Autodesk Fusion 360 part; units mm, degrees
(part 2 of 4)
  line L565 (-143.125, 35.2707) -> (-143.125, 31.2293)
  line L566 (-143.125, 31.2293) -> (-139.625, 29.2085)
  line L567 (-136.125, 31.2293) -> (-136.125, 35.2707)
  line L568 (-152.125, 31.2293) -> (-148.625, 29.2085)
  line L569 (-122.625, 43.065) -> (-126.125, 45.0857)
  line L570 (-126.125, 45.0857) -> (-129.625, 43.065)
  line L571 (-122.625, 39.0235) -> (-122.625, 43.065)
  line L572 (-134.125, 35.2707) -> (-134.125, 31.2293)
  line L573 (-127.125, 31.2293) -> (-127.125, 35.2707)
  line L574 (-129.625, 39.0235) -> (-126.125, 37.0028)
  line L575 (-135.125, 45.0857) -> (-138.625, 43.065)
  line L576 (-131.625, 39.0235) -> (-131.625, 43.065)
  line L577 (-130.625, 37.2915) -> (-134.125, 35.2707)
  line L578 (-130.625, 29.2085) -> (-127.125, 31.2293)
  line L579 (-131.625, 43.065) -> (-135.125, 45.0857)
  line L580 (-138.625, 39.0235) -> (-135.125, 37.0028)
  line L581 (-135.125, 37.0028) -> (-131.625, 39.0235)
  line L582 (-127.125, 35.2707) -> (-130.625, 37.2915)
  line L583 (-129.625, 43.065) -> (-129.625, 39.0235)
  line L584 (-138.625, 43.065) -> (-138.625, 39.0235)
  line L585 (-126.125, 37.0028) -> (-122.625, 39.0235)
  line L586 (-121.625, 37.2915) -> (-125.125, 35.2707)
  line L587 (-118.125, 35.2707) -> (-121.625, 37.2915)
  line L588 (-121.625, 29.2085) -> (-118.125, 31.2293)
  line L589 (-125.125, 35.2707) -> (-125.125, 31.2293)
  line L590 (-125.125, 31.2293) -> (-121.625, 29.2085)
  line L591 (-118.125, 31.2293) -> (-118.125, 35.2707)
  line L592 (-134.125, 31.2293) -> (-130.625, 29.2085)
  line L593 (-104.625, 43.065) -> (-108.125, 45.0857)
  line L594 (-108.125, 45.0857) -> (-111.625, 43.065)
  line L595 (-104.625, 39.0235) -> (-104.625, 43.065)
  line L596 (-116.125, 35.2707) -> (-116.125, 31.2293)
  line L597 (-109.125, 31.2293) -> (-109.125, 35.2707)
  line L598 (-111.625, 39.0235) -> (-108.125, 37.0028)
  line L599 (-117.125, 45.0857) -> (-120.625, 43.065)
  line L600 (-113.625, 39.0235) -> (-113.625, 43.065)
  line L601 (-112.625, 37.2915) -> (-116.125, 35.2707)
  line L602 (-112.625, 29.2085) -> (-109.125, 31.2293)
  line L603 (-113.625, 43.065) -> (-117.125, 45.0857)
  line L604 (-120.625, 39.0235) -> (-117.125, 37.0028)
  line L605 (-117.125, 37.0028) -> (-113.625, 39.0235)
  line L606 (-109.125, 35.2707) -> (-112.625, 37.2915)
  line L607 (-111.625, 43.065) -> (-111.625, 39.0235)
  line L608 (-120.625, 43.065) -> (-120.625, 39.0235)
  line L609 (-108.125, 37.0028) -> (-104.625, 39.0235)
  line L610 (-103.625, 37.2915) -> (-107.125, 35.2707)
  line L611 (-100.125, 35.2707) -> (-103.625, 37.2915)
  line L612 (-103.625, 29.2085) -> (-100.125, 31.2293)
  line L613 (-107.125, 35.2707) -> (-107.125, 31.2293)
  line L614 (-107.125, 31.2293) -> (-103.625, 29.2085)
  line L615 (-100.125, 31.2293) -> (-100.125, 35.2707)
  line L616 (-116.125, 31.2293) -> (-112.625, 29.2085)
  line L617 (-86.625, 43.065) -> (-90.125, 45.0857)
  line L618 (-90.125, 45.0857) -> (-93.625, 43.065)
  line L619 (-86.625, 39.0235) -> (-86.625, 43.065)
  line L620 (-98.125, 35.2707) -> (-98.125, 31.2293)
  line L621 (-91.125, 31.2293) -> (-91.125, 35.2707)
  line L622 (-93.625, 39.0235) -> (-90.125, 37.0028)
  line L623 (-99.125, 45.0857) -> (-102.625, 43.065)
  line L624 (-95.625, 39.0235) -> (-95.625, 43.065)
  line L625 (-94.625, 37.2915) -> (-98.125, 35.2707)
  line L626 (-94.625, 29.2085) -> (-91.125, 31.2293)
  line L627 (-95.625, 43.065) -> (-99.125, 45.0857)
  line L628 (-102.625, 39.0235) -> (-99.125, 37.0028)
  line L629 (-99.125, 37.0028) -> (-95.625, 39.0235)
  line L630 (-91.125, 35.2707) -> (-94.625, 37.2915)
  line L631 (-93.625, 43.065) -> (-93.625, 39.0235)
  line L632 (-102.625, 43.065) -> (-102.625, 39.0235)
  line L633 (-90.125, 37.0028) -> (-86.625, 39.0235)
  line L634 (-85.625, 37.2915) -> (-89.125, 35.2707)
  line L635 (-82.125, 35.2707) -> (-85.625, 37.2915)
  line L636 (-85.625, 29.2085) -> (-82.125, 31.2293)
  line L637 (-89.125, 35.2707) -> (-89.125, 31.2293)
  line L638 (-89.125, 31.2293) -> (-85.625, 29.2085)
  line L639 (-82.125, 31.2293) -> (-82.125, 35.2707)
  line L640 (-98.125, 31.2293) -> (-94.625, 29.2085)
  line L641 (-50.625, 43.065) -> (-54.125, 45.0857)
  line L642 (-54.125, 45.0857) -> (-57.625, 43.065)
  line L643 (-50.625, 39.0235) -> (-50.625, 43.065)
  line L644 (-62.125, 35.2707) -> (-62.125, 31.2293)
  line L645 (-55.125, 31.2293) -> (-55.125, 35.2707)
  line L646 (-57.625, 39.0235) -> (-54.125, 37.0028)
  line L647 (-63.125, 45.0857) -> (-66.625, 43.065)
  line L648 (-59.625, 39.0235) -> (-59.625, 43.065)
  line L649 (-58.625, 37.2915) -> (-62.125, 35.2707)
  line L650 (-58.625, 29.2085) -> (-55.125, 31.2293)
  line L651 (-59.625, 43.065) -> (-63.125, 45.0857)
  line L652 (-66.625, 39.0235) -> (-63.125, 37.0028)
  line L653 (-63.125, 37.0028) -> (-59.625, 39.0235)
  line L654 (-55.125, 35.2707) -> (-58.625, 37.2915)
  line L655 (-57.625, 43.065) -> (-57.625, 39.0235)
  line L656 (-66.625, 43.065) -> (-66.625, 39.0235)
  line L657 (-54.125, 37.0028) -> (-50.625, 39.0235)
  line L658 (-49.625, 37.2915) -> (-53.125, 35.2707)
  line L659 (-46.125, 35.2707) -> (-49.625, 37.2915)
  line L660 (-49.625, 29.2085) -> (-46.125, 31.2293)
  line L661 (-53.125, 35.2707) -> (-53.125, 31.2293)
  line L662 (-53.125, 31.2293) -> (-49.625, 29.2085)
  line L663 (-46.125, 31.2293) -> (-46.125, 35.2707)
  line L664 (-62.125, 31.2293) -> (-58.625, 29.2085)
  line L665 (-32.625, 43.065) -> (-36.125, 45.0857)
  line L666 (-36.125, 45.0857) -> (-39.625, 43.065)
  line L667 (-32.625, 39.0235) -> (-32.625, 43.065)
  line L668 (-44.125, 35.2707) -> (-44.125, 31.2293)
  line L669 (-37.125, 31.2293) -> (-37.125, 35.2707)
  line L670 (-39.625, 39.0235) -> (-36.125, 37.0028)
  line L671 (-45.125, 45.0857) -> (-48.625, 43.065)
  line L672 (-41.625, 39.0235) -> (-41.625, 43.065)
  line L673 (-40.625, 37.2915) -> (-44.125, 35.2707)
  line L674 (-40.625, 29.2085) -> (-37.125, 31.2293)
  line L675 (-41.625, 43.065) -> (-45.125, 45.0857)
  line L676 (-48.625, 39.0235) -> (-45.125, 37.0028)
  line L677 (-45.125, 37.0028) -> (-41.625, 39.0235)
  line L678 (-37.125, 35.2707) -> (-40.625, 37.2915)
  line L679 (-39.625, 43.065) -> (-39.625, 39.0235)
  line L680 (-48.625, 43.065) -> (-48.625, 39.0235)
  line L681 (-36.125, 37.0028) -> (-32.625, 39.0235)
  line L682 (-31.625, 37.2915) -> (-35.125, 35.2707)
  line L683 (-28.125, 35.2707) -> (-31.625, 37.2915)
  line L684 (-31.625, 29.2085) -> (-28.125, 31.2293)
  line L685 (-35.125, 35.2707) -> (-35.125, 31.2293)
  line L686 (-35.125, 31.2293) -> (-31.625, 29.2085)
  line L687 (-28.125, 31.2293) -> (-28.125, 35.2707)
  line L688 (-44.125, 31.2293) -> (-40.625, 29.2085)
  line L689 (-14.625, 43.065) -> (-18.125, 45.0857)
  line L690 (-18.125, 45.0857) -> (-21.625, 43.065)
  line L691 (-14.625, 39.0235) -> (-14.625, 43.065)
  line L692 (-26.125, 35.2707) -> (-26.125, 31.2293)
  line L693 (-19.125, 31.2293) -> (-19.125, 35.2707)
  line L694 (-21.625, 39.0235) -> (-18.125, 37.0028)
  line L695 (-27.125, 45.0857) -> (-30.625, 43.065)
  line L696 (-23.625, 39.0235) -> (-23.625, 43.065)
  line L697 (-22.625, 37.2915) -> (-26.125, 35.2707)
  line L698 (-22.625, 29.2085) -> (-19.125, 31.2293)
  line L699 (-23.625, 43.065) -> (-27.125, 45.0857)
  line L700 (-30.625, 39.0235) -> (-27.125, 37.0028)
  line L701 (-27.125, 37.0028) -> (-23.625, 39.0235)
  line L702 (-19.125, 35.2707) -> (-22.625, 37.2915)
  line L703 (-21.625, 43.065) -> (-21.625, 39.0235)
  line L704 (-30.625, 43.065) -> (-30.625, 39.0235)
  line L705 (-18.125, 37.0028) -> (-14.625, 39.0235)
  line L706 (-13.625, 37.2915) -> (-17.125, 35.2707)
  line L707 (-10.125, 35.2707) -> (-13.625, 37.2915)
  line L708 (-13.625, 29.2085) -> (-10.125, 31.2293)
  line L709 (-17.125, 35.2707) -> (-17.125, 31.2293)
  line L710 (-17.125, 31.2293) -> (-13.625, 29.2085)
  line L711 (-10.125, 31.2293) -> (-10.125, 35.2707)
  line L712 (-26.125, 31.2293) -> (-22.625, 29.2085)
  line L713 (3.375, 43.065) -> (-0.125, 45.0857)
  line L714 (-0.125, 45.0857) -> (-3.625, 43.065)
  line L715 (3.375, 39.0235) -> (3.375, 43.065)
  line L716 (-8.125, 35.2707) -> (-8.125, 31.2293)
  line L717 (-1.125, 31.2293) -> (-1.125, 35.2707)
  line L718 (-3.625, 39.0235) -> (-0.125, 37.0028)
  line L719 (-9.125, 45.0857) -> (-12.625, 43.065)
  line L720 (-5.625, 39.0235) -> (-5.625, 43.065)
  line L721 (-4.625, 37.2915) -> (-8.125, 35.2707)
  line L722 (-4.625, 29.2085) -> (-1.125, 31.2293)
  line L723 (-5.625, 43.065) -> (-9.125, 45.0857)
  line L724 (-12.625, 39.0235) -> (-9.125, 37.0028)
  line L725 (-9.125, 37.0028) -> (-5.625, 39.0235)
  line L726 (-1.125, 35.2707) -> (-4.625, 37.2915)
  line L727 (-3.625, 43.065) -> (-3.625, 39.0235)
  line L728 (-12.625, 43.065) -> (-12.625, 39.0235)
  line L729 (-0.125, 37.0028) -> (3.375, 39.0235)
  line L730 (4.375, 37.2915) -> (0.875, 35.2707)
  line L731 (7.875, 35.2707) -> (4.375, 37.2915)
  line L732 (4.375, 29.2085) -> (7.875, 31.2293)
  line L733 (0.875, 35.2707) -> (0.875, 31.2293)
  line L734 (0.875, 31.2293) -> (4.375, 29.2085)
  line L735 (7.875, 31.2293) -> (7.875, 35.2707)
  line L736 (-8.125, 31.2293) -> (-4.625, 29.2085)
  line L737 (21.375, 43.065) -> (17.875, 45.0857)
  line L738 (17.875, 45.0857) -> (14.375, 43.065)
  line L739 (21.375, 39.0235) -> (21.375, 43.065)
  line L740 (9.875, 35.2707) -> (9.875, 31.2293)
  line L741 (16.875, 31.2293) -> (16.875, 35.2707)
  line L742 (14.375, 39.0235) -> (17.875, 37.0028)
  line L743 (8.875, 45.0857) -> (5.375, 43.065)
  line L744 (12.375, 39.0235) -> (12.375, 43.065)
  line L745 (13.375, 37.2915) -> (9.875, 35.2707)
  line L746 (13.375, 29.2085) -> (16.875, 31.2293)
  line L747 (12.375, 43.065) -> (8.875, 45.0857)
  line L748 (5.375, 39.0235) -> (8.875, 37.0028)
  line L749 (8.875, 37.0028) -> (12.375, 39.0235)
  line L750 (16.875, 35.2707) -> (13.375, 37.2915)
  line L751 (14.375, 43.065) -> (14.375, 39.0235)
  line L752 (5.375, 43.065) -> (5.375, 39.0235)
  line L753 (17.875, 37.0028) -> (21.375, 39.0235)
  line L754 (22.375, 37.2915) -> (18.875, 35.2707)
  line L755 (25.875, 35.2707) -> (22.375, 37.2915)
  line L756 (22.375, 29.2085) -> (25.875, 31.2293)
  line L757 (18.875, 35.2707) -> (18.875, 31.2293)
  line L758 (18.875, 31.2293) -> (22.375, 29.2085)
  line L759 (25.875, 31.2293) -> (25.875, 35.2707)
  line L760 (9.875, 31.2293) -> (13.375, 29.2085)
  line L761 (-140.625, 58.942) -> (-144.125, 60.9627)
  line L762 (-144.125, 60.9627) -> (-147.625, 58.942)
  line L763 (-140.625, 54.9005) -> (-140.625, 58.942)
  line L764 (-152.125, 51.1477) -> (-152.125, 47.1063)
  line L765 (-145.125, 47.1063) -> (-145.125, 51.1477)
  line L766 (-147.625, 54.9005) -> (-144.125, 52.8798)
  line L767 (-153.125, 60.9627) -> (-156.625, 58.942)
  line L768 (-149.625, 54.9005) -> (-149.625, 58.942)
  line L769 (-148.625, 53.1685) -> (-152.125, 51.1477)
  line L770 (-148.625, 45.0855) -> (-145.125, 47.1063)
  line L771 (-149.625, 58.942) -> (-153.125, 60.9627)
  line L772 (-156.625, 54.9005) -> (-153.125, 52.8798)
  line L773 (-153.125, 52.8798) -> (-149.625, 54.9005)
  line L774 (-145.125, 51.1477) -> (-148.625, 53.1685)
  line L775 (-147.625, 58.942) -> (-147.625, 54.9005)
  line L776 (-156.625, 58.942) -> (-156.625, 54.9005)
  line L777 (-144.125, 52.8798) -> (-140.625, 54.9005)
  line L778 (-139.625, 53.1685) -> (-143.125, 51.1477)
  line L779 (-136.125, 51.1477) -> (-139.625, 53.1685)
  line L780 (-139.625, 45.0855) -> (-136.125, 47.1063)
  line L781 (-143.125, 51.1477) -> (-143.125, 47.1063)
  line L782 (-143.125, 47.1063) -> (-139.625, 45.0855)
  line L783 (-136.125, 47.1063) -> (-136.125, 51.1477)
  line L784 (-152.125, 47.1063) -> (-148.625, 45.0855)
  line L785 (-122.625, 58.942) -> (-126.125, 60.9627)
  line L786 (-126.125, 60.9627) -> (-129.625, 58.942)
  line L787 (-122.625, 54.9005) -> (-122.625, 58.942)
  line L788 (-134.125, 51.1477) -> (-134.125, 47.1063)
  line L789 (-127.125, 47.1063) -> (-127.125, 51.1477)
  line L790 (-129.625, 54.9005) -> (-126.125, 52.8798)
  line L791 (-135.125, 60.9627) -> (-138.625, 58.942)
  line L792 (-131.625, 54.9005) -> (-131.625, 58.942)
  line L793 (-130.625, 53.1685) -> (-134.125, 51.1477)
  line L794 (-130.625, 45.0855) -> (-127.125, 47.1063)
  line L795 (-131.625, 58.942) -> (-135.125, 60.9627)
  line L796 (-138.625, 54.9005) -> (-135.125, 52.8798)
  line L797 (-135.125, 52.8798) -> (-131.625, 54.9005)
  line L798 (-127.125, 51.1477) -> (-130.625, 53.1685)
  line L799 (-129.625, 58.942) -> (-129.625, 54.9005)
  line L800 (-138.625, 58.942) -> (-138.625, 54.9005)
  line L801 (-126.125, 52.8798) -> (-122.625, 54.9005)
  line L802 (-121.625, 53.1685) -> (-125.125, 51.1477)
  line L803 (-118.125, 51.1477) -> (-121.625, 53.1685)
  line L804 (-121.625, 45.0855) -> (-118.125, 47.1063)
  line L805 (-125.125, 51.1477) -> (-125.125, 47.1063)
  line L806 (-125.125, 47.1063) -> (-121.625, 45.0855)
  line L807 (-118.125, 47.1063) -> (-118.125, 51.1477)
  line L808 (-134.125, 47.1063) -> (-130.625, 45.0855)
  line L809 (-104.625, 58.942) -> (-108.125, 60.9627)
  line L810 (-108.125, 60.9627) -> (-111.625, 58.942)
  line L811 (-104.625, 54.9005) -> (-104.625, 58.942)
  line L812 (-116.125, 51.1477) -> (-116.125, 47.1063)
  line L813 (-109.125, 47.1063) -> (-109.125, 51.1477)
  line L814 (-111.625, 54.9005) -> (-108.125, 52.8798)
  line L815 (-117.125, 60.9627) -> (-120.625, 58.942)
  line L816 (-113.625, 54.9005) -> (-113.625, 58.942)
  line L817 (-112.625, 53.1685) -> (-116.125, 51.1477)
  line L818 (-112.625, 45.0855) -> (-109.125, 47.1063)
  line L819 (-113.625, 58.942) -> (-117.125, 60.9627)
  line L820 (-120.625, 54.9005) -> (-117.125, 52.8798)
  line L821 (-117.125, 52.8798) -> (-113.625, 54.9005)
  line L822 (-109.125, 51.1477) -> (-112.625, 53.1685)
  line L823 (-111.625, 58.942) -> (-111.625, 54.9005)
  line L824 (-120.625, 58.942) -> (-120.625, 54.9005)
  line L825 (-108.125, 52.8798) -> (-104.625, 54.9005)
  line L826 (-103.625, 53.1685) -> (-107.125, 51.1477)
  line L827 (-100.125, 51.1477) -> (-103.625, 53.1685)
  line L828 (-103.625, 45.0855) -> (-100.125, 47.1063)
  line L829 (-107.125, 51.1477) -> (-107.125, 47.1063)
  line L830 (-107.125, 47.1063) -> (-103.625, 45.0855)
  line L831 (-100.125, 47.1063) -> (-100.125, 51.1477)
  line L832 (-116.125, 47.1063) -> (-112.625, 45.0855)
  line L833 (-86.625, 58.942) -> (-90.125, 60.9627)
  line L834 (-90.125, 60.9627) -> (-93.625, 58.942)
  line L835 (-86.625, 54.9005) -> (-86.625, 58.942)
  line L836 (-98.125, 51.1477) -> (-98.125, 47.1063)
  line L837 (-91.125, 47.1063) -> (-91.125, 51.1477)
  line L838 (-93.625, 54.9005) -> (-90.125, 52.8798)
  line L839 (-99.125, 60.9627) -> (-102.625, 58.942)
  line L840 (-95.625, 54.9005) -> (-95.625, 58.942)
  line L841 (-94.625, 53.1685) -> (-98.125, 51.1477)
  line L842 (-94.625, 45.0855) -> (-91.125, 47.1063)
  line L843 (-95.625, 58.942) -> (-99.125, 60.9627)
  line L844 (-102.625, 54.9005) -> (-99.125, 52.8798)
  line L845 (-99.125, 52.8798) -> (-95.625, 54.9005)
  line L846 (-91.125, 51.1477) -> (-94.625, 53.1685)
  line L847 (-93.625, 58.942) -> (-93.625, 54.9005)
  line L848 (-102.625, 58.942) -> (-102.625, 54.9005)
  line L849 (-90.125, 52.8798) -> (-86.625, 54.9005)
  line L850 (-85.625, 53.1685) -> (-89.125, 51.1477)
  line L851 (-82.125, 51.1477) -> (-85.625, 53.1685)
  line L852 (-85.625, 45.0855) -> (-82.125, 47.1063)
  line L853 (-89.125, 51.1477) -> (-89.125, 47.1063)
  line L854 (-89.125, 47.1063) -> (-85.625, 45.0855)
  line L855 (-82.125, 47.1063) -> (-82.125, 51.1477)
  line L856 (-98.125, 47.1063) -> (-94.625, 45.0855)
  line L857 (-68.625, 58.942) -> (-72.125, 60.9627)
  line L858 (-72.125, 60.9627) -> (-75.625, 58.942)
  line L859 (-68.625, 54.9005) -> (-68.625, 58.942)
  line L860 (-80.125, 51.1477) -> (-80.125, 47.1063)
  line L861 (-73.125, 47.1063) -> (-73.125, 51.1477)
  line L862 (-75.625, 54.9005) -> (-72.125, 52.8798)
  line L863 (-81.125, 60.9627) -> (-84.625, 58.942)
  line L864 (-77.625, 54.9005) -> (-77.625, 58.942)
  line L865 (-76.625, 53.1685) -> (-80.125, 51.1477)
  line L866 (-76.625, 45.0855) -> (-73.125, 47.1063)
  line L867 (-77.625, 58.942) -> (-81.125, 60.9627)
  line L868 (-84.625, 54.9005) -> (-81.125, 52.8798)
  line L869 (-81.125, 52.8798) -> (-77.625, 54.9005)
  line L870 (-73.125, 51.1477) -> (-76.625, 53.1685)
  line L871 (-75.625, 58.942) -> (-75.625, 54.9005)
  line L872 (-84.625, 58.942) -> (-84.625, 54.9005)
  line L873 (-72.125, 52.8798) -> (-68.625, 54.9005)
  line L874 (-67.625, 53.1685) -> (-71.125, 51.1477)
  line L875 (-64.125, 51.1477) -> (-67.625, 53.1685)
  line L876 (-67.625, 45.0855) -> (-64.125, 47.1063)
  line L877 (-71.125, 51.1477) -> (-71.125, 47.1063)
  line L878 (-71.125, 47.1063) -> (-67.625, 45.0855)
  line L879 (-64.125, 47.1063) -> (-64.125, 51.1477)
  line L880 (-80.125, 47.1063) -> (-76.625, 45.0855)
  line L881 (-50.625, 58.942) -> (-54.125, 60.9627)
  line L882 (-54.125, 60.9627) -> (-57.625, 58.942)
  line L883 (-50.625, 54.9005) -> (-50.625, 58.942)
  line L884 (-62.125, 51.1477) -> (-62.125, 47.1063)
  line L885 (-55.125, 47.1063) -> (-55.125, 51.1477)
  line L886 (-57.625, 54.9005) -> (-54.125, 52.8798)
  line L887 (-63.125, 60.9627) -> (-66.625, 58.942)
  line L888 (-59.625, 54.9005) -> (-59.625, 58.942)
  line L889 (-58.625, 53.1685) -> (-62.125, 51.1477)
  line L890 (-58.625, 45.0855) -> (-55.125, 47.1063)
  line L891 (-59.625, 58.942) -> (-63.125, 60.9627)
  line L892 (-66.625, 54.9005) -> (-63.125, 52.8798)
  line L893 (-63.125, 52.8798) -> (-59.625, 54.9005)
  line L894 (-55.125, 51.1477) -> (-58.625, 53.1685)
  line L895 (-57.625, 58.942) -> (-57.625, 54.9005)
  line L896 (-66.625, 58.942) -> (-66.625, 54.9005)
  line L897 (-54.125, 52.8798) -> (-50.625, 54.9005)
  line L898 (-49.625, 53.1685) -> (-53.125, 51.1477)
  line L899 (-46.125, 51.1477) -> (-49.625, 53.1685)
  line L900 (-49.625, 45.0855) -> (-46.125, 47.1063)
  line L901 (-53.125, 51.1477) -> (-53.125, 47.1063)
  line L902 (-53.125, 47.1063) -> (-49.625, 45.0855)
  line L903 (-46.125, 47.1063) -> (-46.125, 51.1477)
  line L904 (-62.125, 47.1063) -> (-58.625, 45.0855)
  line L905 (-32.625, 58.942) -> (-36.125, 60.9627)
  line L906 (-36.125, 60.9627) -> (-39.625, 58.942)
  line L907 (-32.625, 54.9005) -> (-32.625, 58.942)
  line L908 (-44.125, 51.1477) -> (-44.125, 47.1063)
  line L909 (-37.125, 47.1063) -> (-37.125, 51.1477)
  line L910 (-39.625, 54.9005) -> (-36.125, 52.8798)
  line L911 (-45.125, 60.9627) -> (-48.625, 58.942)
  line L912 (-41.625, 54.9005) -> (-41.625, 58.942)
  line L913 (-40.625, 53.1685) -> (-44.125, 51.1477)
  line L914 (-40.625, 45.0855) -> (-37.125, 47.1063)
  line L915 (-41.625, 58.942) -> (-45.125, 60.9627)
  line L916 (-48.625, 54.9005) -> (-45.125, 52.8798)
  line L917 (-45.125, 52.8798) -> (-41.625, 54.9005)
  line L918 (-37.125, 51.1477) -> (-40.625, 53.1685)
  line L919 (-39.625, 58.942) -> (-39.625, 54.9005)
  line L920 (-48.625, 58.942) -> (-48.625, 54.9005)
  line L921 (-36.125, 52.8798) -> (-32.625, 54.9005)
  line L922 (-31.625, 53.1685) -> (-35.125, 51.1477)
  line L923 (-28.125, 51.1477) -> (-31.625, 53.1685)
  line L924 (-31.625, 45.0855) -> (-28.125, 47.1063)
  line L925 (-35.125, 51.1477) -> (-35.125, 47.1063)
  line L926 (-35.125, 47.1063) -> (-31.625, 45.0855)
  line L927 (-28.125, 47.1063) -> (-28.125, 51.1477)
  line L928 (-44.125, 47.1063) -> (-40.625, 45.0855)
  line L929 (-14.625, 58.942) -> (-18.125, 60.9627)
  line L930 (-18.125, 60.9627) -> (-21.625, 58.942)
  line L931 (-14.625, 54.9005) -> (-14.625, 58.942)
  line L932 (-26.125, 51.1477) -> (-26.125, 47.1063)
  line L933 (-19.125, 47.1063) -> (-19.125, 51.1477)
  line L934 (-21.625, 54.9005) -> (-18.125, 52.8798)
  line L935 (-27.125, 60.9627) -> (-30.625, 58.942)
  line L936 (-23.625, 54.9005) -> (-23.625, 58.942)
  line L937 (-22.625, 53.1685) -> (-26.125, 51.1477)
  line L938 (-22.625, 45.0855) -> (-19.125, 47.1063)
  line L939 (-23.625, 58.942) -> (-27.125, 60.9627)
  line L940 (-30.625, 54.9005) -> (-27.125, 52.8798)
  line L941 (-27.125, 52.8798) -> (-23.625, 54.9005)
  line L942 (-19.125, 51.1477) -> (-22.625, 53.1685)
  line L943 (-21.625, 58.942) -> (-21.625, 54.9005)
  line L944 (-30.625, 58.942) -> (-30.625, 54.9005)
  line L945 (-18.125, 52.8798) -> (-14.625, 54.9005)
  line L946 (-13.625, 53.1685) -> (-17.125, 51.1477)
  line L947 (-10.125, 51.1477) -> (-13.625, 53.1685)
  line L948 (-13.625, 45.0855) -> (-10.125, 47.1063)
  line L949 (-17.125, 51.1477) -> (-17.125, 47.1063)
  line L950 (-17.125, 47.1063) -> (-13.625, 45.0855)
  line L951 (-10.125, 47.1063) -> (-10.125, 51.1477)
  line L952 (-26.125, 47.1063) -> (-22.625, 45.0855)
  line L953 (3.375, 58.942) -> (-0.125, 60.9627)
  line L954 (-0.125, 60.9627) -> (-3.625, 58.942)
  line L955 (3.375, 54.9005) -> (3.375, 58.942)
  line L956 (-8.125, 51.1477) -> (-8.125, 47.1063)
  line L957 (-1.125, 47.1063) -> (-1.125, 51.1477)
  line L958 (-3.625, 54.9005) -> (-0.125, 52.8798)
  line L959 (-9.125, 60.9627) -> (-12.625, 58.942)
  line L960 (-5.625, 54.9005) -> (-5.625, 58.942)
  line L961 (-4.625, 53.1685) -> (-8.125, 51.1477)
  line L962 (-4.625, 45.0855) -> (-1.125, 47.1063)
  line L963 (-5.625, 58.942) -> (-9.125, 60.9627)
  line L964 (-12.625, 54.9005) -> (-9.125, 52.8798)
  line L965 (-9.125, 52.8798) -> (-5.625, 54.9005)
  line L966 (-1.125, 51.1477) -> (-4.625, 53.1685)
  line L967 (-3.625, 58.942) -> (-3.625, 54.9005)
  line L968 (-12.625, 58.942) -> (-12.625, 54.9005)
  line L969 (-0.125, 52.8798) -> (3.375, 54.9005)
  line L970 (4.375, 53.1685) -> (0.875, 51.1477)
  line L971 (7.875, 51.1477) -> (4.375, 53.1685)
  line L972 (4.375, 45.0855) -> (7.875, 47.1063)
  line L973 (0.875, 51.1477) -> (0.875, 47.1063)
  line L974 (0.875, 47.1063) -> (4.375, 45.0855)
  line L975 (7.875, 47.1063) -> (7.875, 51.1477)
  line L976 (-8.125, 47.1063) -> (-4.625, 45.0855)
  line L977 (21.375, 58.942) -> (17.875, 60.9627)
  line L978 (17.875, 60.9627) -> (14.375, 58.942)
  line L979 (21.375, 54.9005) -> (21.375, 58.942)
  line L980 (9.875, 51.1477) -> (9.875, 47.1063)
  line L981 (16.875, 47.1063) -> (16.875, 51.1477)
  line L982 (14.375, 54.9005) -> (17.875, 52.8798)
  line L983 (8.875, 60.9627) -> (5.375, 58.942)
  line L984 (12.375, 54.9005) -> (12.375, 58.942)
  line L985 (13.375, 53.1685) -> (9.875, 51.1477)
  line L986 (13.375, 45.0855) -> (16.875, 47.1063)
  line L987 (12.375, 58.942) -> (8.875, 60.9627)
  line L988 (5.375, 54.9005) -> (8.875, 52.8798)
  line L989 (8.875, 52.8798) -> (12.375, 54.9005)
  line L990 (16.875, 51.1477) -> (13.375, 53.1685)
  line L991 (14.375, 58.942) -> (14.375, 54.9005)
  line L992 (5.375, 58.942) -> (5.375, 54.9005)
  line L993 (17.875, 52.8798) -> (21.375, 54.9005)
  line L994 (22.375, 53.1685) -> (18.875, 51.1477)
  line L995 (25.875, 51.1477) -> (22.375, 53.1685)
  line L996 (22.375, 45.0855) -> (25.875, 47.1063)
  line L997 (18.875, 51.1477) -> (18.875, 47.1063)
  line L998 (18.875, 47.1063) -> (22.375, 45.0855)
  line L999 (25.875, 47.1063) -> (25.875, 51.1477)
  line L1000 (9.875, 47.1063) -> (13.375, 45.0855)
  line L1001 (-140.625, 74.819) -> (-144.125, 76.8397)
  line L1002 (-144.125, 76.8397) -> (-147.625, 74.819)
  line L1003 (-140.625, 70.7775) -> (-140.625, 74.819)
  line L1004 (-152.125, 67.0247) -> (-152.125, 62.9833)
  line L1005 (-145.125, 62.9833) -> (-145.125, 67.0247)
  line L1006 (-147.625, 70.7775) -> (-144.125, 68.7568)
  line L1007 (-153.125, 76.8397) -> (-156.625, 74.819)
  line L1008 (-149.625, 70.7775) -> (-149.625, 74.819)
  line L1009 (-148.625, 69.0455) -> (-152.125, 67.0247)
  line L1010 (-148.625, 60.9625) -> (-145.125, 62.9833)
  line L1011 (-149.625, 74.819) -> (-153.125, 76.8397)
  line L1012 (-156.625, 70.7775) -> (-153.125, 68.7568)
  line L1013 (-153.125, 68.7568) -> (-149.625, 70.7775)
  line L1014 (-145.125, 67.0247) -> (-148.625, 69.0455)
  line L1015 (-147.625, 74.819) -> (-147.625, 70.7775)
  line L1016 (-156.625, 74.819) -> (-156.625, 70.7775)
  line L1017 (-144.125, 68.7568) -> (-140.625, 70.7775)
  line L1018 (-139.625, 69.0455) -> (-143.125, 67.0247)
  line L1019 (-136.125, 67.0247) -> (-139.625, 69.0455)
  line L1020 (-139.625, 60.9625) -> (-136.125, 62.9833)
  line L1021 (-143.125, 67.0247) -> (-143.125, 62.9833)
  line L1022 (-143.125, 62.9833) -> (-139.625, 60.9625)
  line L1023 (-136.125, 62.9833) -> (-136.125, 67.0247)
  line L1024 (-152.125, 62.9833) -> (-148.625, 60.9625)
  line L1025 (-122.625, 74.819) -> (-126.125, 76.8397)
  line L1026 (-126.125, 76.8397) -> (-129.625, 74.819)
  line L1027 (-122.625, 70.7775) -> (-122.625, 74.819)
  line L1028 (-134.125, 67.0247) -> (-134.125, 62.9833)
  line L1029 (-127.125, 62.9833) -> (-127.125, 67.0247)
  line L1030 (-129.625, 70.7775) -> (-126.125, 68.7568)
  line L1031 (-135.125, 76.8397) -> (-138.625, 74.819)
  line L1032 (-131.625, 70.7775) -> (-131.625, 74.819)
  line L1033 (-130.625, 69.0455) -> (-134.125, 67.0247)
  line L1034 (-130.625, 60.9625) -> (-127.125, 62.9833)
  line L1035 (-131.625, 74.819) -> (-135.125, 76.8397)
  line L1036 (-138.625, 70.7775) -> (-135.125, 68.7568)
  line L1037 (-135.125, 68.7568) -> (-131.625, 70.7775)
  line L1038 (-127.125, 67.0247) -> (-130.625, 69.0455)
  line L1039 (-129.625, 74.819) -> (-129.625, 70.7775)
  line L1040 (-138.625, 74.819) -> (-138.625, 70.7775)
  line L1041 (-126.125, 68.7568) -> (-122.625, 70.7775)
  line L1042 (-121.625, 69.0455) -> (-125.125, 67.0247)
  line L1043 (-118.125, 67.0247) -> (-121.625, 69.0455)
  line L1044 (-121.625, 60.9625) -> (-118.125, 62.9833)
  line L1045 (-125.125, 67.0247) -> (-125.125, 62.9833)
  line L1046 (-125.125, 62.9833) -> (-121.625, 60.9625)
  line L1047 (-118.125, 62.9833) -> (-118.125, 67.0247)
  line L1048 (-134.125, 62.9833) -> (-130.625, 60.9625)
  line L1049 (-104.625, 74.819) -> (-108.125, 76.8397)
  line L1050 (-108.125, 76.8397) -> (-111.625, 74.819)
  line L1051 (-104.625, 70.7775) -> (-104.625, 74.819)
  line L1052 (-116.125, 67.0247) -> (-116.125, 62.9833)
  line L1053 (-109.125, 62.9833) -> (-109.125, 67.0247)
  line L1054 (-111.625, 70.7775) -> (-108.125, 68.7568)
  line L1055 (-117.125, 76.8397) -> (-120.625, 74.819)
  line L1056 (-113.625, 70.7775) -> (-113.625, 74.819)
  line L1057 (-112.625, 69.0455) -> (-116.125, 67.0247)
  line L1058 (-112.625, 60.9625) -> (-109.125, 62.9833)
  line L1059 (-113.625, 74.819) -> (-117.125, 76.8397)
  line L1060 (-120.625, 70.7775) -> (-117.125, 68.7568)
  line L1061 (-117.125, 68.7568) -> (-113.625, 70.7775)
  line L1062 (-109.125, 67.0247) -> (-112.625, 69.0455)
  line L1063 (-111.625, 74.819) -> (-111.625, 70.7775)
  line L1064 (-120.625, 74.819) -> (-120.625, 70.7775)
  line L1065 (-108.125, 68.7568) -> (-104.625, 70.7775)
  line L1066 (-103.625, 69.0455) -> (-107.125, 67.0247)
  line L1067 (-100.125, 67.0247) -> (-103.625, 69.0455)
  line L1068 (-103.625, 60.9625) -> (-100.125, 62.9833)
  line L1069 (-107.125, 67.0247) -> (-107.125, 62.9833)
  line L1070 (-107.125, 62.9833) -> (-103.625, 60.9625)
  line L1071 (-100.125, 62.9833) -> (-100.125, 67.0247)
  line L1072 (-116.125, 62.9833) -> (-112.625, 60.9625)
  line L1073 (-86.625, 74.819) -> (-90.125, 76.8397)
  line L1074 (-90.125, 76.8397) -> (-93.625, 74.819)
  line L1075 (-86.625, 70.7775) -> (-86.625, 74.819)
  line L1076 (-98.125, 67.0247) -> (-98.125, 62.9833)
  line L1077 (-91.125, 62.9833) -> (-91.125, 67.0247)
  line L1078 (-93.625, 70.7775) -> (-90.125, 68.7568)
  line L1079 (-99.125, 76.8397) -> (-102.625, 74.819)
  line L1080 (-95.625, 70.7775) -> (-95.625, 74.819)
  line L1081 (-94.625, 69.0455) -> (-98.125, 67.0247)
  line L1082 (-94.625, 60.9625) -> (-91.125, 62.9833)
  line L1083 (-95.625, 74.819) -> (-99.125, 76.8397)
  line L1084 (-102.625, 70.7775) -> (-99.125, 68.7568)
  line L1085 (-99.125, 68.7568) -> (-95.625, 70.7775)
  line L1086 (-91.125, 67.0247) -> (-94.625, 69.0455)
  line L1087 (-93.625, 74.819) -> (-93.625, 70.7775)
  line L1088 (-102.625, 74.819) -> (-102.625, 70.7775)
  line L1089 (-90.125, 68.7568) -> (-86.625, 70.7775)
  line L1090 (-85.625, 69.0455) -> (-89.125, 67.0247)
  line L1091 (-82.125, 67.0247) -> (-85.625, 69.0455)
  line L1092 (-85.625, 60.9625) -> (-82.125, 62.9833)
  line L1093 (-89.125, 67.0247) -> (-89.125, 62.9833)
  line L1094 (-89.125, 62.9833) -> (-85.625, 60.9625)
  line L1095 (-82.125, 62.9833) -> (-82.125, 67.0247)
  line L1096 (-98.125, 62.9833) -> (-94.625, 60.9625)
  line L1097 (-68.625, 74.819) -> (-72.125, 76.8397)
  line L1098 (-72.125, 76.8397) -> (-75.625, 74.819)
  line L1099 (-68.625, 70.7775) -> (-68.625, 74.819)
  line L1100 (-80.125, 67.0247) -> (-80.125, 62.9833)
  line L1101 (-73.125, 62.9833) -> (-73.125, 67.0247)
  line L1102 (-75.625, 70.7775) -> (-72.125, 68.7568)
  line L1103 (-81.125, 76.8397) -> (-84.625, 74.819)
  line L1104 (-77.625, 70.7775) -> (-77.625, 74.819)
  line L1105 (-76.625, 69.0455) -> (-80.125, 67.0247)
  line L1106 (-76.625, 60.9625) -> (-73.125, 62.9833)
  line L1107 (-77.625, 74.819) -> (-81.125, 76.8397)
  line L1108 (-84.625, 70.7775) -> (-81.125, 68.7568)
  line L1109 (-81.125, 68.7568) -> (-77.625, 70.7775)
  line L1110 (-73.125, 67.0247) -> (-76.625, 69.0455)
  line L1111 (-75.625, 74.819) -> (-75.625, 70.7775)
  line L1112 (-84.625, 74.819) -> (-84.625, 70.7775)
  line L1113 (-72.125, 68.7568) -> (-68.625, 70.7775)
  line L1114 (-67.625, 69.0455) -> (-71.125, 67.0247)
  line L1115 (-64.125, 67.0247) -> (-67.625, 69.0455)
  line L1116 (-67.625, 60.9625) -> (-64.125, 62.9833)
  line L1117 (-71.125, 67.0247) -> (-71.125, 62.9833)
  line L1118 (-71.125, 62.9833) -> (-67.625, 60.9625)
  line L1119 (-64.125, 62.9833) -> (-64.125, 67.0247)
  line L1120 (-80.125, 62.9833) -> (-76.625, 60.9625)
  line L1121 (-50.625, 74.819) -> (-54.125, 76.8397)
  line L1122 (-54.125, 76.8397) -> (-57.625, 74.819)
  line L1123 (-50.625, 70.7775) -> (-50.625, 74.819)
  line L1124 (-62.125, 67.0247) -> (-62.125, 62.9833)
  line L1125 (-55.125, 62.9833) -> (-55.125, 67.0247)
  line L1126 (-57.625, 70.7775) -> (-54.125, 68.7568)
  line L1127 (-63.125, 76.8397) -> (-66.625, 74.819)
  line L1128 (-59.625, 70.7775) -> (-59.625, 74.819)
  line L1129 (-58.625, 69.0455) -> (-62.125, 67.0247)
  line L1130 (-58.625, 60.9625) -> (-55.125, 62.9833)
  line L1131 (-59.625, 74.819) -> (-63.125, 76.8397)
  line L1132 (-66.625, 70.7775) -> (-63.125, 68.7568)
  line L1133 (-63.125, 68.7568) -> (-59.625, 70.7775)
  line L1134 (-55.125, 67.0247) -> (-58.625, 69.0455)
  line L1135 (-57.625, 74.819) -> (-57.625, 70.7775)
  line L1136 (-66.625, 74.819) -> (-66.625, 70.7775)
  line L1137 (-54.125, 68.7568) -> (-50.625, 70.7775)
  line L1138 (-49.625, 69.0455) -> (-53.125, 67.0247)
  line L1139 (-46.125, 67.0247) -> (-49.625, 69.0455)
  line L1140 (-49.625, 60.9625) -> (-46.125, 62.9833)
  line L1141 (-53.125, 67.0247) -> (-53.125, 62.9833)
  line L1142 (-53.125, 62.9833) -> (-49.625, 60.9625)
  line L1143 (-46.125, 62.9833) -> (-46.125, 67.0247)
  line L1144 (-62.125, 62.9833) -> (-58.625, 60.9625)
  line L1145 (-32.625, 74.819) -> (-36.125, 76.8397)
  line L1146 (-36.125, 76.8397) -> (-39.625, 74.819)
  line L1147 (-32.625, 70.7775) -> (-32.625, 74.819)
  line L1148 (-44.125, 67.0247) -> (-44.125, 62.9833)
  line L1149 (-37.125, 62.9833) -> (-37.125, 67.0247)
  line L1150 (-39.625, 70.7775) -> (-36.125, 68.7568)
  line L1151 (-45.125, 76.8397) -> (-48.625, 74.819)
  line L1152 (-41.625, 70.7775) -> (-41.625, 74.819)
  line L1153 (-40.625, 69.0455) -> (-44.125, 67.0247)
  line L1154 (-40.625, 60.9625) -> (-37.125, 62.9833)
  line L1155 (-41.625, 74.819) -> (-45.125, 76.8397)
  line L1156 (-48.625, 70.7775) -> (-45.125, 68.7568)
  line L1157 (-45.125, 68.7568) -> (-41.625, 70.7775)
  line L1158 (-37.125, 67.0247) -> (-40.625, 69.0455)
  line L1159 (-39.625, 74.819) -> (-39.625, 70.7775)
  line L1160 (-48.625, 74.819) -> (-48.625, 70.7775)
  line L1161 (-36.125, 68.7568) -> (-32.625, 70.7775)
  line L1162 (-31.625, 69.0455) -> (-35.125, 67.0247)
  line L1163 (-28.125, 67.0247) -> (-31.625, 69.0455)
  line L1164 (-31.625, 60.9625) -> (-28.125, 62.9833)
  line L1165 (-35.125, 67.0247) -> (-35.125, 62.9833)
  line L1166 (-35.125, 62.9833) -> (-31.625, 60.9625)
  line L1167 (-28.125, 62.9833) -> (-28.125, 67.0247)
  line L1168 (-44.125, 62.9833) -> (-40.625, 60.9625)
  line L1169 (-14.625, 74.819) -> (-18.125, 76.8397)
  line L1170 (-18.125, 76.8397) -> (-21.625, 74.819)
  line L1171 (-14.625, 70.7775) -> (-14.625, 74.819)
  line L1172 (-26.125, 67.0247) -> (-26.125, 62.9833)
  line L1173 (-19.125, 62.9833) -> (-19.125, 67.0247)
  line L1174 (-21.625, 70.7775) -> (-18.125, 68.7568)
  line L1175 (-27.125, 76.8397) -> (-30.625, 74.819)
  line L1176 (-23.625, 70.7775) -> (-23.625, 74.819)
  line L1177 (-22.625, 69.0455) -> (-26.125, 67.0247)
  line L1178 (-22.625, 60.9625) -> (-19.125, 62.9833)
  line L1179 (-23.625, 74.819) -> (-27.125, 76.8397)
  line L1180 (-30.625, 70.7775) -> (-27.125, 68.7568)
  line L1181 (-27.125, 68.7568) -> (-23.625, 70.7775)
  line L1182 (-19.125, 67.0247) -> (-22.625, 69.0455)
  line L1183 (-21.625, 74.819) -> (-21.625, 70.7775)
  line L1184 (-30.625, 74.819) -> (-30.625, 70.7775)
  line L1185 (-18.125, 68.7568) -> (-14.625, 70.7775)
  line L1186 (-13.625, 69.0455) -> (-17.125, 67.0247)
  line L1187 (-10.125, 67.0247) -> (-13.625, 69.0455)
  line L1188 (-13.625, 60.9625) -> (-10.125, 62.9833)
  line L1189 (-17.125, 67.0247) -> (-17.125, 62.9833)
  line L1190 (-17.125, 62.9833) -> (-13.625, 60.9625)
  line L1191 (-10.125, 62.9833) -> (-10.125, 67.0247)
  line L1192 (-26.125, 62.9833) -> (-22.625, 60.9625)
  line L1193 (3.375, 74.819) -> (-0.125, 76.8397)
  line L1194 (-0.125, 76.8397) -> (-3.625, 74.819)
  line L1195 (3.375, 70.7775) -> (3.375, 74.819)
  line L1196 (-8.125, 67.0247) -> (-8.125, 62.9833)
  line L1197 (-1.125, 62.9833) -> (-1.125, 67.0247)
  line L1198 (-3.625, 70.7775) -> (-0.125, 68.7568)
  line L1199 (-9.125, 76.8397) -> (-12.625, 74.819)
  line L1200 (-5.625, 70.7775) -> (-5.625, 74.819)
  line L1201 (-4.625, 69.0455) -> (-8.125, 67.0247)
  line L1202 (-4.625, 60.9625) -> (-1.125, 62.9833)
  line L1203 (-5.625, 74.819) -> (-9.125, 76.8397)
  line L1204 (-12.625, 70.7775) -> (-9.125, 68.7568)
  line L1205 (-9.125, 68.7568) -> (-5.625, 70.7775)
  line L1206 (-1.125, 67.0247) -> (-4.625, 69.0455)
  line L1207 (-3.625, 74.819) -> (-3.625, 70.7775)
  line L1208 (-12.625, 74.819) -> (-12.625, 70.7775)
  line L1209 (-0.125, 68.7568) -> (3.375, 70.7775)
  line L1210 (4.375, 69.0455) -> (0.875, 67.0247)
  line L1211 (7.875, 67.0247) -> (4.375, 69.0455)
  line L1212 (4.375, 60.9625) -> (7.875, 62.9833)
  line L1213 (0.875, 67.0247) -> (0.875, 62.9833)
  line L1214 (0.875, 62.9833) -> (4.375, 60.9625)
  line L1215 (7.875, 62.9833) -> (7.875, 67.0247)
  line L1216 (-8.125, 62.9833) -> (-4.625, 60.9625)
  line L1217 (21.375, 74.819) -> (17.875, 76.8397)
  line L1218 (17.875, 76.8397) -> (14.375, 74.819)
  line L1219 (21.375, 70.7775) -> (21.375, 74.819)
  line L1220 (9.875, 67.0247) -> (9.875, 62.9833)
  line L1221 (16.875, 62.9833) -> (16.875, 67.0247)
  line L1222 (14.375, 70.7775) -> (17.875, 68.7568)
  line L1223 (8.875, 76.8397) -> (5.375, 74.819)
  line L1224 (12.375, 70.7775) -> (12.375, 74.819)
  line L1225 (13.375, 69.0455) -> (9.875, 67.0247)
  line L1226 (13.375, 60.9625) -> (16.875, 62.9833)
  line L1227 (12.375, 74.819) -> (8.875, 76.8397)
  line L1228 (5.375, 70.7775) -> (8.875, 68.7568)
  line L1229 (8.875, 68.7568) -> (12.375, 70.7775)
  line L1230 (16.875, 67.0247) -> (13.375, 69.0455)
  line L1231 (14.375, 74.819) -> (14.375, 70.7775)
  line L1232 (5.375, 74.819) -> (5.375, 70.7775)
  line L1233 (17.875, 68.7568) -> (21.375, 70.7775)
  line L1234 (22.375, 69.0455) -> (18.875, 67.0247)
  line L1235 (25.875, 67.0247) -> (22.375, 69.0455)
  line L1236 (22.375, 60.9625) -> (25.875, 62.9833)
  line L1237 (18.875, 67.0247) -> (18.875, 62.9833)
  line L1238 (18.875, 62.9833) -> (22.375, 60.9625)
  line L1239 (25.875, 62.9833) -> (25.875, 67.0247)
  line L1240 (9.875, 62.9833) -> (13.375, 60.9625)
  line L1241 (-140.625, 90.696) -> (-144.125, 92.7167)
  line L1242 (-144.125, 92.7167) -> (-147.625, 90.696)
  line L1243 (-140.625, 86.6545) -> (-140.625, 90.696)
  line L1244 (-152.125, 82.9017) -> (-152.125, 78.8603)
  line L1245 (-145.125, 78.8603) -> (-145.125, 82.9017)
  line L1246 (-147.625, 86.6545) -> (-144.125, 84.6338)
  line L1247 (-153.125, 92.7167) -> (-156.625, 90.696)
  line L1248 (-149.625, 86.6545) -> (-149.625, 90.696)
  line L1249 (-148.625, 84.9225) -> (-152.125, 82.9017)
  line L1250 (-148.625, 76.8395) -> (-145.125, 78.8603)
  line L1251 (-149.625, 90.696) -> (-153.125, 92.7167)
  line L1252 (-156.625, 86.6545) -> (-153.125, 84.6338)
  line L1253 (-153.125, 84.6338) -> (-149.625, 86.6545)
  line L1254 (-145.125, 82.9017) -> (-148.625, 84.9225)
  line L1255 (-147.625, 90.696) -> (-147.625, 86.6545)
  line L1256 (-156.625, 90.696) -> (-156.625, 86.6545)
  line L1257 (-144.125, 84.6338) -> (-140.625, 86.6545)
  line L1258 (-139.625, 84.9225) -> (-143.125, 82.9017)
  line L1259 (-136.125, 82.9017) -> (-139.625, 84.9225)
  line L1260 (-139.625, 76.8395) -> (-136.125, 78.8603)
  line L1261 (-143.125, 82.9017) -> (-143.125, 78.8603)
  line L1262 (-143.125, 78.8603) -> (-139.625, 76.8395)
  line L1263 (-136.125, 78.8603) -> (-136.125, 82.9017)
  line L1264 (-152.125, 78.8603) -> (-148.625, 76.8395)
  line L1265 (-122.625, 90.696) -> (-126.125, 92.7167)
  line L1266 (-126.125, 92.7167) -> (-129.625, 90.696)
  line L1267 (-122.625, 86.6545) -> (-122.625, 90.696)
  line L1268 (-134.125, 82.9017) -> (-134.125, 78.8603)
  line L1269 (-127.125, 78.8603) -> (-127.125, 82.9017)
  line L1270 (-129.625, 86.6545) -> (-126.125, 84.6338)
  line L1271 (-135.125, 92.7167) -> (-138.625, 90.696)
  line L1272 (-131.625, 86.6545) -> (-131.625, 90.696)
  line L1273 (-130.625, 84.9225) -> (-134.125, 82.9017)
  line L1274 (-130.625, 76.8395) -> (-127.125, 78.8603)
  line L1275 (-131.625, 90.696) -> (-135.125, 92.7167)
  line L1276 (-138.625, 86.6545) -> (-135.125, 84.6338)
  line L1277 (-135.125, 84.6338) -> (-131.625, 86.6545)
  line L1278 (-127.125, 82.9017) -> (-130.625, 84.9225)
  line L1279 (-129.625, 90.696) -> (-129.625, 86.6545)
  line L1280 (-138.625, 90.696) -> (-138.625, 86.6545)
  line L1281 (-126.125, 84.6338) -> (-122.625, 86.6545)
  line L1282 (-121.625, 84.9225) -> (-125.125, 82.9017)
  line L1283 (-118.125, 82.9017) -> (-121.625, 84.9225)
  line L1284 (-121.625, 76.8395) -> (-118.125, 78.8603)
  line L1285 (-125.125, 82.9017) -> (-125.125, 78.8603)
  line L1286 (-125.125, 78.8603) -> (-121.625, 76.8395)
  line L1287 (-118.125, 78.8603) -> (-118.125, 82.9017)
  line L1288 (-134.125, 78.8603) -> (-130.625, 76.8395)
  line L1289 (-104.625, 90.696) -> (-108.125, 92.7167)
  line L1290 (-108.125, 92.7167) -> (-111.625, 90.696)
  line L1291 (-104.625, 86.6545) -> (-104.625, 90.696)
  line L1292 (-116.125, 82.9017) -> (-116.125, 78.8603)
  line L1293 (-109.125, 78.8603) -> (-109.125, 82.9017)
  line L1294 (-111.625, 86.6545) -> (-108.125, 84.6338)
  line L1295 (-117.125, 92.7167) -> (-120.625, 90.696)
  line L1296 (-113.625, 86.6545) -> (-113.625, 90.696)
  line L1297 (-112.625, 84.9225) -> (-116.125, 82.9017)
  line L1298 (-112.625, 76.8395) -> (-109.125, 78.8603)
  line L1299 (-113.625, 90.696) -> (-117.125, 92.7167)
  line L1300 (-120.625, 86.6545) -> (-117.125, 84.6338)
  line L1301 (-117.125, 84.6338) -> (-113.625, 86.6545)
  line L1302 (-109.125, 82.9017) -> (-112.625, 84.9225)
  line L1303 (-111.625, 90.696) -> (-111.625, 86.6545)
  line L1304 (-120.625, 90.696) -> (-120.625, 86.6545)
  line L1305 (-108.125, 84.6338) -> (-104.625, 86.6545)
  line L1306 (-103.625, 84.9225) -> (-107.125, 82.9017)
  line L1307 (-100.125, 82.9017) -> (-103.625, 84.9225)
  line L1308 (-103.625, 76.8395) -> (-100.125, 78.8603)
  line L1309 (-107.125, 82.9017) -> (-107.125, 78.8603)
  line L1310 (-107.125, 78.8603) -> (-103.625, 76.8395)
  line L1311 (-100.125, 78.8603) -> (-100.125, 82.9017)
  line L1312 (-116.125, 78.8603) -> (-112.625, 76.8395)
  line L1313 (-86.625, 90.696) -> (-90.125, 92.7167)
  line L1314 (-90.125, 92.7167) -> (-93.625, 90.696)
  line L1315 (-86.625, 86.6545) -> (-86.625, 90.696)
  line L1316 (-98.125, 82.9017) -> (-98.125, 78.8603)
  line L1317 (-91.125, 78.8603) -> (-91.125, 82.9017)
  line L1318 (-93.625, 86.6545) -> (-90.125, 84.6338)
  line L1319 (-99.125, 92.7167) -> (-102.625, 90.696)
  line L1320 (-95.625, 86.6545) -> (-95.625, 90.696)
  line L1321 (-94.625, 84.9225) -> (-98.125, 82.9017)
  line L1322 (-94.625, 76.8395) -> (-91.125, 78.8603)
  line L1323 (-95.625, 90.696) -> (-99.125, 92.7167)
  line L1324 (-102.625, 86.6545) -> (-99.125, 84.6338)
  line L1325 (-99.125, 84.6338) -> (-95.625, 86.6545)
  line L1326 (-91.125, 82.9017) -> (-94.625, 84.9225)
  line L1327 (-93.625, 90.696) -> (-93.625, 86.6545)
  line L1328 (-102.625, 90.696) -> (-102.625, 86.6545)
  line L1329 (-90.125, 84.6338) -> (-86.625, 86.6545)
  line L1330 (-85.625, 84.9225) -> (-89.125, 82.9017)
  line L1331 (-82.125, 82.9017) -> (-85.625, 84.9225)
  line L1332 (-85.625, 76.8395) -> (-82.125, 78.8603)
  line L1333 (-89.125, 82.9017) -> (-89.125, 78.8603)
  line L1334 (-89.125, 78.8603) -> (-85.625, 76.8395)
  line L1335 (-82.125, 78.8603) -> (-82.125, 82.9017)
  line L1336 (-98.125, 78.8603) -> (-94.625, 76.8395)
  line L1337 (-68.625, 90.696) -> (-72.125, 92.7167)
  line L1338 (-72.125, 92.7167) -> (-75.625, 90.696)
  line L1339 (-68.625, 86.6545) -> (-68.625, 90.696)
  line L1340 (-80.125, 82.9017) -> (-80.125, 78.8603)
  line L1341 (-73.125, 78.8603) -> (-73.125, 82.9017)
  line L1342 (-75.625, 86.6545) -> (-72.125, 84.6338)
  line L1343 (-81.125, 92.7167) -> (-84.625, 90.696)
  line L1344 (-77.625, 86.6545) -> (-77.625, 90.696)
  line L1345 (-76.625, 84.9225) -> (-80.125, 82.9017)
  line L1346 (-76.625, 76.8395) -> (-73.125, 78.8603)
  line L1347 (-77.625, 90.696) -> (-81.125, 92.7167)
  line L1348 (-84.625, 86.6545) -> (-81.125, 84.6338)
  line L1349 (-81.125, 84.6338) -> (-77.625, 86.6545)
  line L1350 (-73.125, 82.9017) -> (-76.625, 84.9225)
  line L1351 (-75.625, 90.696) -> (-75.625, 86.6545)
  line L1352 (-84.625, 90.696) -> (-84.625, 86.6545)
  line L1353 (-72.125, 84.6338) -> (-68.625, 86.6545)
  line L1354 (-67.625, 84.9225) -> (-71.125, 82.9017)
  line L1355 (-64.125, 82.9017) -> (-67.625, 84.9225)
  line L1356 (-67.625, 76.8395) -> (-64.125, 78.8603)
  line L1357 (-71.125, 82.9017) -> (-71.125, 78.8603)
  line L1358 (-71.125, 78.8603) -> (-67.625, 76.8395)
  line L1359 (-64.125, 78.8603) -> (-64.125, 82.9017)
  line L1360 (-80.125, 78.8603) -> (-76.625, 76.8395)
  line L1361 (-50.625, 90.696) -> (-54.125, 92.7167)
  line L1362 (-54.125, 92.7167) -> (-57.625, 90.696)
  line L1363 (-50.625, 86.6545) -> (-50.625, 90.696)
  line L1364 (-62.125, 82.9017) -> (-62.125, 78.8603)
  line L1365 (-55.125, 78.8603) -> (-55.125, 82.9017)
  line L1366 (-57.625, 86.6545) -> (-54.125, 84.6338)
  line L1367 (-63.125, 92.7167) -> (-66.625, 90.696)
  line L1368 (-59.625, 86.6545) -> (-59.625, 90.696)
  line L1369 (-58.625, 84.9225) -> (-62.125, 82.9017)
  line L1370 (-58.625, 76.8395) -> (-55.125, 78.8603)
  line L1371 (-59.625, 90.696) -> (-63.125, 92.7167)
  line L1372 (-66.625, 86.6545) -> (-63.125, 84.6338)
  line L1373 (-63.125, 84.6338) -> (-59.625, 86.6545)
  line L1374 (-55.125, 82.9017) -> (-58.625, 84.9225)
  line L1375 (-57.625, 90.696) -> (-57.625, 86.6545)
  line L1376 (-66.625, 90.696) -> (-66.625, 86.6545)
  line L1377 (-54.125, 84.6338) -> (-50.625, 86.6545)
  line L1378 (-49.625, 84.9225) -> (-53.125, 82.9017)
  line L1379 (-46.125, 82.9017) -> (-49.625, 84.9225)
  line L1380 (-49.625, 76.8395) -> (-46.125, 78.8603)
  line L1381 (-53.125, 82.9017) -> (-53.125, 78.8603)
  line L1382 (-53.125, 78.8603) -> (-49.625, 76.8395)
  line L1383 (-46.125, 78.8603) -> (-46.125, 82.9017)
  line L1384 (-62.125, 78.8603) -> (-58.625, 76.8395)
  line L1385 (-32.625, 90.696) -> (-36.125, 92.7167)
  line L1386 (-36.125, 92.7167) -> (-39.625, 90.696)
  line L1387 (-32.625, 86.6545) -> (-32.625, 90.696)
  line L1388 (-44.125, 82.9017) -> (-44.125, 78.8603)
  line L1389 (-37.125, 78.8603) -> (-37.125, 82.9017)
  line L1390 (-39.625, 86.6545) -> (-36.125, 84.6338)
  line L1391 (-45.125, 92.7167) -> (-48.625, 90.696)
  line L1392 (-41.625, 86.6545) -> (-41.625, 90.696)
  line L1393 (-40.625, 84.9225) -> (-44.125, 82.9017)
  line L1394 (-40.625, 76.8395) -> (-37.125, 78.8603)
  line L1395 (-41.625, 90.696) -> (-45.125, 92.7167)
  line L1396 (-48.625, 86.6545) -> (-45.125, 84.6338)
  line L1397 (-45.125, 84.6338) -> (-41.625, 86.6545)
  line L1398 (-37.125, 82.9017) -> (-40.625, 84.9225)
  line L1399 (-39.625, 90.696) -> (-39.625, 86.6545)
  line L1400 (-48.625, 90.696) -> (-48.625, 86.6545)
  line L1401 (-36.125, 84.6338) -> (-32.625, 86.6545)
  line L1402 (-31.625, 84.9225) -> (-35.125, 82.9017)
  line L1403 (-28.125, 82.9017) -> (-31.625, 84.9225)
  line L1404 (-31.625, 76.8395) -> (-28.125, 78.8603)
  line L1405 (-35.125, 82.9017) -> (-35.125, 78.8603)
  line L1406 (-35.125, 78.8603) -> (-31.625, 76.8395)
  line L1407 (-28.125, 78.8603) -> (-28.125, 82.9017)
  line L1408 (-44.125, 78.8603) -> (-40.625, 76.8395)
  line L1409 (-14.625, 90.696) -> (-18.125, 92.7167)
  line L1410 (-18.125, 92.7167) -> (-21.625, 90.696)
  line L1411 (-14.625, 86.6545) -> (-14.625, 90.696)
  line L1412 (-26.125, 82.9017) -> (-26.125, 78.8603)
  line L1413 (-19.125, 78.8603) -> (-19.125, 82.9017)
  line L1414 (-21.625, 86.6545) -> (-18.125, 84.6338)
  line L1415 (-27.125, 92.7167) -> (-30.625, 90.696)
  line L1416 (-23.625, 86.6545) -> (-23.625, 90.696)
  line L1417 (-22.625, 84.9225) -> (-26.125, 82.9017)
  line L1418 (-22.625, 76.8395) -> (-19.125, 78.8603)
  line L1419 (-23.625, 90.696) -> (-27.125, 92.7167)
  line L1420 (-30.625, 86.6545) -> (-27.125, 84.6338)
  line L1421 (-27.125, 84.6338) -> (-23.625, 86.6545)
  line L1422 (-19.125, 82.9017) -> (-22.625, 84.9225)
  line L1423 (-21.625, 90.696) -> (-21.625, 86.6545)
  line L1424 (-30.625, 90.696) -> (-30.625, 86.6545)
  line L1425 (-18.125, 84.6338) -> (-14.625, 86.6545)
  line L1426 (-13.625, 84.9225) -> (-17.125, 82.9017)
  line L1427 (-10.125, 82.9017) -> (-13.625, 84.9225)
  line L1428 (-13.625, 76.8395) -> (-10.125, 78.8603)
  line L1429 (-17.125, 82.9017) -> (-17.125, 78.8603)
  line L1430 (-17.125, 78.8603) -> (-13.625, 76.8395)
  line L1431 (-10.125, 78.8603) -> (-10.125, 82.9017)
  line L1432 (-26.125, 78.8603) -> (-22.625, 76.8395)
  line L1433 (3.375, 90.696) -> (-0.125, 92.7167)
  line L1434 (-0.125, 92.7167) -> (-3.625, 90.696)
  line L1435 (3.375, 86.6545) -> (3.375, 90.696)
  line L1436 (-8.125, 82.9017) -> (-8.125, 78.8603)
  line L1437 (-1.125, 78.8603) -> (-1.125, 82.9017)
  line L1438 (-3.625, 86.6545) -> (-0.125, 84.6338)
  line L1439 (-9.125, 92.7167) -> (-12.625, 90.696)
  line L1440 (-5.625, 86.6545) -> (-5.625, 90.696)
  line L1441 (-4.625, 84.9225) -> (-8.125, 82.9017)
  line L1442 (-4.625, 76.8395) -> (-1.125, 78.8603)
  line L1443 (-5.625, 90.696) -> (-9.125, 92.7167)
  line L1444 (-12.625, 86.6545) -> (-9.125, 84.6338)
  line L1445 (-9.125, 84.6338) -> (-5.625, 86.6545)
  line L1446 (-1.125, 82.9017) -> (-4.625, 84.9225)
  line L1447 (-3.625, 90.696) -> (-3.625, 86.6545)
  line L1448 (-12.625, 90.696) -> (-12.625, 86.6545)
  line L1449 (-0.125, 84.6338) -> (3.375, 86.6545)
  line L1450 (4.375, 84.9225) -> (0.875, 82.9017)
  line L1451 (7.875, 82.9017) -> (4.375, 84.9225)
  line L1452 (4.375, 76.8395) -> (7.875, 78.8603)
  line L1453 (0.875, 82.9017) -> (0.875, 78.8603)
  line L1454 (0.875, 78.8603) -> (4.375, 76.8395)
  line L1455 (7.875, 78.8603) -> (7.875, 82.9017)
  line L1456 (-8.125, 78.8603) -> (-4.625, 76.8395)
  line L1457 (21.375, 90.696) -> (17.875, 92.7167)
  line L1458 (17.875, 92.7167) -> (14.375, 90.696)
  line L1459 (21.375, 86.6545) -> (21.375, 90.696)
  line L1460 (9.875, 82.9017) -> (9.875, 78.8603)
  line L1461 (16.875, 78.8603) -> (16.875, 82.9017)
  line L1462 (14.375, 86.6545) -> (17.875, 84.6338)
  line L1463 (8.875, 92.7167) -> (5.375, 90.696)
  line L1464 (12.375, 86.6545) -> (12.375, 90.696)
  line L1465 (13.375, 84.9225) -> (9.875, 82.9017)
  line L1466 (13.375, 76.8395) -> (16.875, 78.8603)
  line L1467 (12.375, 90.696) -> (8.875, 92.7167)
  line L1468 (5.375, 86.6545) -> (8.875, 84.6338)
  line L1469 (8.875, 84.6338) -> (12.375, 86.6545)
  line L1470 (16.875, 82.9017) -> (13.375, 84.9225)
  line L1471 (14.375, 90.696) -> (14.375, 86.6545)
  line L1472 (5.375, 90.696) -> (5.375, 86.6545)
  line L1473 (17.875, 84.6338) -> (21.375, 86.6545)
  line L1474 (22.375, 84.9225) -> (18.875, 82.9017)
  line L1475 (25.875, 82.9017) -> (22.375, 84.9225)
  line L1476 (22.375, 76.8395) -> (25.875, 78.8603)
  line L1477 (18.875, 82.9017) -> (18.875, 78.8603)
  line L1478 (18.875, 78.8603) -> (22.375, 76.8395)
  line L1479 (25.875, 78.8603) -> (25.875, 82.9017)
  line L1480 (9.875, 78.8603) -> (13.375, 76.8395)
  line L1481 (-2.25, 60) -> (-151, 60)
  line L1482 (-151, 60) -> (-151, 58)
  line L1483 (-151, 58) -> (-2.25, 58)
  line L1484 (-2.25, 58) -> (-2.25, 60)
  line L1485 (-2.25, 6.5) -> (-2.25, 6.315)
  point P0 (-76.625, 33.25)
  point P1 (-67.625, 33.25)
  point P2 (-72.125, 41.0442)
  point P3 (-81.125, 41.0442)
  point P4 (-153.125, 9.2902)
  point P5 (-144.125, 9.2902)
  point P6 (-139.625, 1.496)
  point P7 (-148.625, 1.496)
  point P8 (-135.125, 9.2902)
  point P9 (-126.125, 9.2902)
  point P10 (-121.625, 1.496)
  point P11 (-130.625, 1.496)
  point P12 (-117.125, 9.2902)
  point P13 (-108.125, 9.2902)
  point P14 (-103.625, 1.496)
  point P15 (-112.625, 1.496)
  point P16 (-99.125, 9.2902)
  point P17 (-90.125, 9.2902)
  point P18 (-85.625, 1.496)
  point P19 (-94.625, 1.496)
  point P20 (-81.125, 9.2902)
  point P21 (-72.125, 9.2902)
  point P22 (-67.625, 1.496)
  point P23 (-76.625, 1.496)
  point P24 (-63.125, 9.2902)
  point P25 (-54.125, 9.2902)
  point P26 (-49.625, 1.496)
  point P27 (-58.625, 1.496)
  point P28 (-45.125, 9.2902)
  point P29 (-36.125, 9.2902)
  point P30 (-31.625, 1.496)